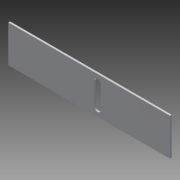
# Autodesk Inventor part: GE_13030
Saved by Autodesk Inventor 2013 (Build 170138000, 138)
## iProperties
Created: 2013-01-02
Part Number: GE_13030
Material: Polyethylene, High Density
Document SubType Name: Modeling
Designer: Phillip
Density: 1 g/cm^3
Author: Phillip
Autodesk Inventor part; units mm, degrees
ref_plane "YZ Plane" through (0, 0, 0) normal (1, 0, 0) x (0, 1, 0)
ref_plane "XZ Plane" through (0, 0, 0) normal (0, 1, 0) x (-1, 0, 0)
ref_plane "XY Plane" through (0, 0, 0) normal (0, 0, 1) x (1, 0, 0)
sketch "Sketch1" plane through (0, 0, 0) normal (0, 0, 1) x (1, 0, 0)
  line L0 (0, 0) -> (552.45, 0)
  line L1 (552.45, 0) -> (552.45, 127)
  line L2 (552.45, 127) -> (0, 127)
  line L3 (0, 127) -> (0, 0)
  dimension "d0" = 552.45
  dimension "d1" = 127
  constraints: 8 end point, 2 parallel, 1 horizontal, 1 perpendicular
  measures "d0" distance of L2.end L1.end
  measures "d1" distance of L1.end L0.end
extrude "Extrusion1" add sketch "Sketch1" against normal blind 6.35
sketch "Sketch2" plane through (0, 0, 0) normal (0, 0, 1) x (1, 0, 0)
  line L0 (552.45, 0) -> (552.45, 127) projected
  line L1 (552.45, 127) -> (0, 127) projected
  line L2 (0, 127) -> (0, 0) projected
  line L3 (315.976, 25.4) -> (315.976, 101.6)
  arc A0 (315.976, 101.6) -> (293.624, 101.6) centre (304.8, 101.6) ccw
  line L4 (293.624, 101.6) -> (293.624, 25.4)
  arc A1 (293.624, 25.4) -> (315.976, 25.4) centre (304.8, 25.4) ccw
  point P0 (276.225, 127)
  dimension "d4" = 76.2
  dimension "d6" = 11.176
  dimension "d7" = 247.65
  dimension "d8" = 25.4
  constraints: 4 end point, 4 point on circle, 4 tangent, 2 centre point, 2 parallel, 1 midpoint
  measures "d4" distance of A1.centre A0.centre
  measures "d6" radius of A0
  measures "d7" distance from line of A0.centre L0
  measures "d8" distance from line of L1 A0.centre
extrude "Extrusion2" cut sketch "Sketch2" against normal up to next
body "Solid1"
